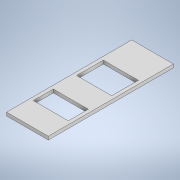
# Autodesk Inventor part: if_case_top
Saved by Autodesk Inventor 2020 (Build 240168000, 168)
## iProperties
Created: 2020-02-14
Part Number: if_case_top
Material: Generic
Document SubType Name: Modeling
Designer: mdjb501
Density: 1 g/cm^3
Appearance: Default
Author: mdjb501
Autodesk Inventor part; units mm, degrees
ref_plane "YZ Plane" through (0, 0, 0) normal (1, 0, 0) x (0, 1, 0)
ref_plane "XZ Plane" through (0, 0, 0) normal (0, 1, 0) x (-1, 0, 0)
ref_plane "XY Plane" through (0, 0, 0) normal (0, 0, 1) x (1, 0, 0)
sketch "Sketch1" plane through (0, 0, 0) normal (0, 1, 0) x (-1, 0, 0)
  line L0 (-6.25, 18.75) -> (6.25, 18.75)
  line L1 (6.25, 18.75) -> (6.25, -18.75)
  line L2 (6.25, -18.75) -> (-6.25, -18.75)
  line L3 (-6.25, -18.75) -> (-6.25, 18.75)
  line L4 (5.25, 18.75) -> (5.25, -18.75)
  line L5 (-5.25, 18.75) -> (-5.25, -18.75)
  line L6 (5.25, 11.75) -> (-5.25, 11.75)
  line L7 (5.25, 5.75) -> (-5.25, 5.75)
  line L8 (5.25, -1.25) -> (-5.25, -1.25)
  line L9 (5.25, -9.25) -> (-5.25, -9.25)
  point P0 (0, 0)
  dimension "d0" = 12.5
  dimension "d1" = 37.5
  constraints: 20 end point, 12 point on line, 3 perpendicular, 2 parallel, 1 horizontal
  measures "d0" distance of L1.end L2.end
  measures "d1" distance of L0.end L1.end
extrude "Extrusion1" add sketch "Sketch1" along normal blind 1 contours L0 L5 L2 L3 | L0 L4 L6 L5 | L0 L1 L2 L4 | L5 L9 L4 L2 | L7 L4 L8 L5
body "Solid1"
